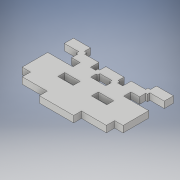
# Autodesk Inventor part: Monster5
Saved by Autodesk Inventor 2019 (Build 230136000, 136)
## iProperties
Created: 2018-12-04
Part Number: Monster5
Material: Generic
Document SubType Name: Modeling
Designer: Administrator
Density: 1 g/cm^3
Appearance: Default
Author: Administrator
Autodesk Inventor part; units mm, degrees
ref_plane "YZ Plane" through (0, 0, 0) normal (1, 0, 0) x (0, 1, 0)
ref_plane "XZ Plane" through (0, 0, 0) normal (0, 1, 0) x (-1, 0, 0)
ref_plane "XY Plane" through (0, 0, 0) normal (0, 0, 1) x (1, 0, 0)
sketch "Sketch1" plane through (0, 0, 0) normal (0, 1, 0) x (-1, 0, 0)
  line L0 (0, 0) -> (426.7814, 0) construction
  line L1 (426.7814, 0) -> (426.7814, -191.0355) construction
  line L2 (426.7814, -191.0355) -> (0, -191.0355) construction
  line L3 (0, -191.0355) -> (0, 0) construction
  line L4 (332.8385, -18.2414) -> (332.8385, -25.9274)
  line L5 (332.8385, -25.9274) -> (308.3392, -25.9274)
  line L6 (308.3392, -25.9274) -> (308.3392, -33.9978)
  line L7 (308.3392, -33.9978) -> (300.0767, -33.9978)
  line L8 (300.0767, -33.9978) -> (300.0767, -59.1696)
  line L9 (300.0767, -59.1696) -> (324.672, -59.1696)
  line L10 (324.672, -59.1696) -> (324.672, -66.3753)
  line L11 (324.672, -66.3753) -> (316.3135, -66.3753)
  line L12 (316.3135, -66.3753) -> (316.3135, -72.5241)
  line L13 (316.3135, -72.5241) -> (314.6458, -72.5241)
  line L14 (314.6458, -72.5241) -> (314.6458, -74.979)
  line L15 (314.6458, -74.979) -> (300.5812, -74.979)
  line L16 (300.5812, -74.979) -> (300.5812, -83.958)
  line L17 (300.5812, -83.958) -> (317.2389, -83.958)
  line L18 (317.2389, -83.958) -> (317.2389, -77.9978)
  line L19 (317.2389, -77.9978) -> (319.6927, -77.9978)
  line L20 (319.6927, -77.9978) -> (319.6927, -75.753)
  line L21 (319.6927, -75.753) -> (333.8192, -75.753)
  line L22 (333.8192, -75.753) -> (333.8192, -67.5016)
  line L23 (333.8192, -67.5016) -> (338.8738, -67.5016)
  line L24 (338.8738, -67.5016) -> (338.8738, -69.7696)
  line L25 (338.8738, -69.7696) -> (340.7167, -69.7696)
  line L26 (340.7167, -69.7696) -> (340.7167, -75.5985)
  line L27 (349.6517, -59.1696) -> (342.2405, -59.1696)
  line L28 (342.2405, -59.1696) -> (342.2405, -64.5393)
  line L29 (342.2405, -64.5393) -> (343.8251, -64.5393)
  line L30 (343.8251, -64.5393) -> (343.8251, -66.7322)
  line L31 (343.8251, -66.7322) -> (349.6517, -66.7322)
  line L32 (325.5834, -43.5764) -> (325.5834, -50.3454)
  line L33 (325.5834, -50.3454) -> (340.7167, -50.3454)
  line L34 (340.7167, -50.3454) -> (340.7167, -43.5764)
  line L35 (340.7167, -43.5764) -> (325.5834, -43.5764)
  line L36 (340.7167, -75.5985) -> (349.6517, -75.5985)
  line L37 (332.8385, -18.2414) -> (349.6517, -18.2414)
  line L38 (366.4649, -18.2414) -> (366.4649, -25.9274)
  line L39 (366.4649, -25.9274) -> (390.9642, -25.9274)
  line L40 (390.9642, -25.9274) -> (390.9642, -33.9978)
  line L41 (390.9642, -33.9978) -> (399.2267, -33.9978)
  line L42 (399.2267, -33.9978) -> (399.2267, -59.1696)
  line L43 (399.2267, -59.1696) -> (374.6314, -59.1696)
  line L44 (374.6314, -59.1696) -> (374.6314, -66.3753)
  line L45 (374.6314, -66.3753) -> (382.9899, -66.3753)
  line L46 (382.9899, -66.3753) -> (382.9899, -72.5241)
  line L47 (382.9899, -72.5241) -> (384.6575, -72.5241)
  line L48 (384.6575, -72.5241) -> (384.6575, -74.979)
  line L49 (384.6575, -74.979) -> (398.7222, -74.979)
  line L50 (398.7222, -74.979) -> (398.7222, -83.958)
  line L51 (398.7222, -83.958) -> (382.0645, -83.958)
  line L52 (382.0645, -83.958) -> (382.0645, -77.9978)
  line L53 (382.0645, -77.9978) -> (379.6107, -77.9978)
  line L54 (379.6107, -77.9978) -> (379.6107, -75.753)
  line L55 (379.6107, -75.753) -> (365.4842, -75.753)
  line L56 (365.4842, -75.753) -> (365.4842, -67.5016)
  line L57 (365.4842, -67.5016) -> (360.4296, -67.5016)
  line L58 (360.4296, -67.5016) -> (360.4296, -69.7696)
  line L59 (360.4296, -69.7696) -> (358.5867, -69.7696)
  line L60 (358.5867, -69.7696) -> (358.5867, -75.5985)
  line L61 (349.6517, -59.1696) -> (357.0629, -59.1696)
  line L62 (357.0629, -59.1696) -> (357.0629, -64.5393)
  line L63 (357.0629, -64.5393) -> (355.4783, -64.5393)
  line L64 (355.4783, -64.5393) -> (355.4783, -66.7322)
  line L65 (355.4783, -66.7322) -> (349.6517, -66.7322)
  line L66 (373.72, -43.5764) -> (373.72, -50.3454)
  line L67 (373.72, -50.3454) -> (358.5867, -50.3454)
  line L68 (358.5867, -50.3454) -> (358.5867, -43.5764)
  line L69 (358.5867, -43.5764) -> (373.72, -43.5764)
  line L70 (358.5867, -75.5985) -> (349.6517, -75.5985)
  line L71 (366.4649, -18.2414) -> (349.6517, -18.2414)
  dimension "d24" = 25.5068
  constraints: 136 end point, 26 perpendicular, 4 point on line, 2 horizontal, 2 vertical, 1 parallel, 2 other
  measures "d24" distance between parallel lines of L8 L32
extrude "Extrusion1" add sketch "Sketch1" along normal blind 6.35
body "Solid1"
